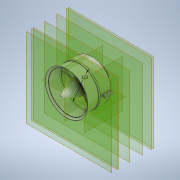
# Autodesk Inventor part: Импеллер
Saved by Autodesk Inventor 2022.1 (Build 261234000, 234)
## iProperties
Created: 2021-12-25
Part Number: Импеллер
Material: Типовые
Document SubType Name: Modeling
Designer: Grigori
Density: 1 g/cm^3
Appearance: По умолчанию
Author: Grigori
Autodesk Inventor part; units mm, degrees
ref_plane "YZ Plane" through (0, 0, 0) normal (1, 0, 0) x (0, 1, 0)
ref_plane "XZ Plane" through (0, 0, 0) normal (0, 1, 0) x (-1, 0, 0)
ref_plane "XY Plane" through (0, 0, 0) normal (0, 0, 1) x (1, 0, 0)
ref_plane "РабПлоскость1" through (-87.3569, 101.8244, 0) normal (0, 0, -1) x (1, 0, 0)
sketch "Эскиз2" plane through (-87.3569, 101.8244, 0) normal (0, 0, -1) x (1, 0, 0)
  circle A0 centre (87.3569, 101.8244) radius 68
  dimension "d1" = 136
  constraints: 1 centre point, 1 coincident
  measures "d1" diameter of A0
ref_plane "РабПлоскость2" through (-87.3569, 101.8244, -5) normal (0, 0, -1) x (1, 0, 0)
sketch "Эскиз3" plane through (-87.3569, 101.8244, -5) normal (0, 0, -1) x (1, 0, 0)
  circle A0 centre (87.3569, 101.8244) radius 62.5
  dimension "d3" = 125
  constraints: 1 centre point, 1 coincident
  measures "d3" diameter of A0
loft "Лофт1" add profiles "Эскиз2", "Эскиз3"
shell "Оболочка1" thickness 1 removed faces 1 at (13.6377, -7.7647, 0)
sketch "Эскиз4" plane through (0, 0, -4) normal (0, 0, 1) x (1, 0, 0)
  circle A0 centre (0, 0) radius 62.1134 projected
extrude "Выдавливание1" cut sketch "Эскиз4" against normal through all
ref_plane "РабПлоскость3" through (-87.3569, 101.8244, -40) normal (0, 0, -1) x (1, 0, 0)
sketch "Эскиз5" plane through (-87.3569, 101.8244, -40) normal (0, 0, -1) x (1, 0, 0)
  circle A0 centre (87.3569, 101.8244) radius 61.5
  dimension "d12" = 123
  constraints: 1 centre point, 1 coincident
  measures "d12" diameter of A0
extrude "Выдавливание2" add sketch "Эскиз5" against normal blind 35
sketch "Эскиз7" plane through (0, 0, -40) normal (0, 0, -1) x (-1, 0, 0)
  circle A0 centre (0, 0) radius 61
  dimension "d15" = 122
  constraints: 1 centre point, 1 coincident
  measures "d15" diameter of A0
extrude "Выдавливание3" cut sketch "Эскиз7" against normal through all
sketch "Эскиз8" plane through (-87.3569, 101.8244, -40) normal (0, 0, -1) x (1, 0, 0)
  circle A0 centre (87.3569, 101.8244) radius 62.5
  circle A1 centre (87.3569, 101.8244) radius 61.5
  dimension "d18" = 125
  constraints: 2 centre point, 2 coincident
  measures "d18" diameter of A0
extrude "Выдавливание4" add sketch "Эскиз8" along normal blind 5
ref_plane "РабПлоскость4" through (-87.3569, 101.8244, -80) normal (0, 0, -1) x (1, 0, 0)
sketch "Эскиз9" plane through (0, 0, -45) normal (0, 0, -1) x (-1, 0, 0)
  circle A0 centre (0, 0) radius 61.5
  dimension "d23" = 123
  constraints: 1 centre point, 1 coincident
  measures "d23" diameter of A0
sketch "Эскиз10" plane through (-87.3569, 101.8244, -80) normal (0, 0, -1) x (1, 0, 0)
  circle A0 centre (87.3569, 101.8244) radius 61.5
  dimension "d24" = 123
  constraints: 1 centre point, 1 coincident
  measures "d24" diameter of A0
loft "Лофт2" add profiles "Эскиз10" section 2 edges at (-61.5, 0, -45)
sketch "Эскиз11" plane through (0, 0, -80) normal (0, 0, -1) x (-1, 0, 0)
  circle A0 centre (0, 0) radius 61
  dimension "d29" = 122
  constraints: 1 centre point, 1 coincident
  measures "d29" diameter of A0
extrude "Выдавливание5" cut sketch "Эскиз11" against normal through all
ref_plane "РабПлоскость6" through (95.8873, -0.0055, 0) normal (0, -1, 0) x (-1, 0, 0)
ref_plane "РабПлоскость8" through (62.5, -0.0055, 0) normal (-1, 0, 0) x (0, 0, -1)
ref_plane "РабПлоскость7" through (0, -0.0055, 0) normal (-1, 0, 0) x (0, 0, -1)
sketch "Эскиз15" plane through (62.5, -0.0055, 0) normal (-1, 0, 0) x (0, 0, -1)
  line L0 (45, -62.5055) -> (45, 62.4945) projected
  line L1 (45, -0.0055) -> (80, -0.0055)
  line L2 (80, 61.4945) -> (80, -61.5055) projected
  line L3 (62.5, -2.0055) -> (75.5, -2.0055)
  line L4 (62.5, -2.0055) -> (49.5, -2.0055)
  line L5 (49.5, -2.0055) -> (49.5, 1.9945)
  line L6 (49.5, 1.9945) -> (75.5, 1.9945)
  line L7 (75.5, 1.9945) -> (75.5, -2.0055)
  point P0 (0, -0.0055)
  dimension "d37" = 13
  dimension "d38" = 13
  dimension "d39" = 4
  constraints: 12 end point, 3 perpendicular, 2 horizontal, 2 midpoint
  measures "d37" distance of L3.start L3.end
  measures "d38" distance of L3.start L4.end
  measures "d39" distance of L4.end L5.end
extrude "Выдавливание6" add sketch "Эскиз15" along normal blind 1.2 and the other way blind 10
sketch "Эскиз17" plane through (61.4675, 2, -49.5) normal (0, 1, 0) x (1, 0, 0)
  line L0 (11.0325, 26) -> (0, 26) projected
  line L1 (11.0325, 0) -> (11.0325, 26)
  circle A0 centre (5.5163, 13) radius 1
  circle A1 centre (5.5163, 3) radius 1
  circle A2 centre (5.5163, 23) radius 1
  point P0 (-61.4675, -49.5)
  dimension "d46" = 2
  dimension "d47" = 2
  dimension "d48" = 2
  constraints: 3 centre point, 2 end point, 1 perpendicular
  measures "d46" diameter of A0
  measures "d47" diameter of A1
  measures "d48" diameter of A2
extrude "Выдавливание7" cut sketch "Эскиз17" against normal through all
mirror "Зеркальное отражение1" about plane through (0, -0.0055, 0) normal (-1, 0, 0) of "Выдавливание6", "Выдавливание7"
ref_plane "РабПлоскость9" through (-87.3569, 101.8244, -110) normal (0, 0, -1) x (1, 0, 0)
sketch "Эскиз18" plane through (-87.3569, 101.8244, -110) normal (0, 0, -1) x (1, 0, 0)
  circle A0 centre (87.3569, 101.8244) radius 24.5
  dimension "d52" = 49
  constraints: 1 centre point, 1 coincident
  measures "d52" diameter of A0
ref_plane "РабПлоскость10" through (-87.3569, 101.8244, -116) normal (0, 0, -1) x (1, 0, 0)
sketch "Эскиз19" plane through (-87.3569, 101.8244, -116) normal (0, 0, -1) x (1, 0, 0)
  circle A0 centre (87.3569, 101.8244) radius 10
  dimension "d54" = 20
  constraints: 1 centre point, 1 coincident
  measures "d54" diameter of A0
loft "Лофт3" add profiles "Эскиз18", "Эскиз19"
sketch "Эскиз20" plane through (0, 0, -110) normal (0, 0, 1) x (1, 0, 0)
  circle A0 centre (0, 0) radius 24.5 projected
sketch "Эскиз22" plane through (-87.3569, 101.8244, -5) normal (0, 0, -1) x (1, 0, 0)
  circle A0 centre (87.3569, 101.8244) radius 61.5
  circle A1 centre (87.3569, 101.8244) radius 61 projected
  circle A2 centre (87.3569, 101.8244) radius 61
  dimension "d59" = 123
  constraints: 2 centre point, 2 coincident
  measures "d59" diameter of A0
extrude "Выдавливание8" add sketch "Эскиз22" along normal blind 75
extrude "Выдавливание9" add sketch "Эскиз20" along normal blind 85
ref_plane "РабПлоскость11" through (-87.3569, 101.8244, 17) normal (0, 0, -1) x (1, 0, 0)
sketch "Эскиз23" plane through (-87.3569, 101.8244, 17) normal (0, 0, -1) x (1, 0, 0)
  circle A0 centre (87.3569, 101.8244) radius 2
  dimension "d65" = 4
  constraints: 1 centre point, 1 coincident
  measures "d65" diameter of A0
sketch "Эскиз24" plane through (0, 0, -25) normal (0, 0, 1) x (1, 0, 0)
  circle A0 centre (0, 0) radius 24.5 projected
loft "Лофт4" add profiles "Эскиз23" section 1 edges at (-24.5, 0, -25)
sketch "Эскиз25" plane through (-87.3569, 101.8244, -40) normal (0, 0, -1) x (1, 0, 0)
  circle A0 centre (87.3569, 101.8244) radius 24.5 projected
  circle A1 centre (87.3569, 101.8244) radius 61 projected
  line L0 (87.3569, 77.3244) -> (87.3569, 77.8106)
  line L1 (87.3569, 40.8244) -> (87.3569, 40.5191)
  line L2 (87.3569, 40.5191) -> (87.8569, 40.5191)
  line L3 (87.8569, 40.5191) -> (87.8569, 77.8106)
  line L4 (87.8569, 77.8106) -> (87.3569, 77.8106)
  line L5 (87.3569, 40.5191) -> (86.8569, 40.5191)
  line L6 (86.8569, 40.5191) -> (86.8569, 77.8106)
  line L7 (86.8569, 77.8106) -> (87.3569, 77.8106)
  point P0 (86.8569, 77.3295)
  point P1 (86.8569, 40.8265)
  point P2 (87.8569, 40.8265)
  point P3 (87.8569, 77.3295)
  dimension "d70" = 0.5
  constraints: 16 end point, 2 perpendicular, 2 vertical, 1 parallel, 4 other
  measures "d70" distance of L1.end L2.end
extrude "Выдавливание10" add sketch "Эскиз25" along normal blind 5 contours A0 L3 A1 L6 picked at (87.468, 65.158)
pattern_circular "Круговой массив1" count 5 over 360 about axis through (0, 0, -110) along (0, 0, 1) of "Выдавливание10"
